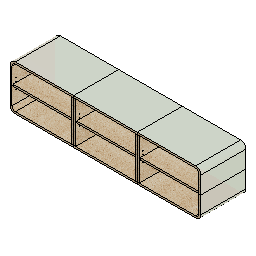
model (Autodesk Fusion 360 design; units mm, degrees)
Autodesk Fusion 360 part; units mm, degrees
note: some values were not read from the file. Chosen so that the rebuilt part matches the saved one: which bodies a step acts on; a side.
sketch "front" plane through (0, 0, 0) normal (0, 1, 0) x (1, 0, 0)
  line L0 (0, 0) -> (1800, 0) construction
  line L1 (1800, 0) -> (1800, -425) construction
  line L2 (1800, -425) -> (0, -425) construction
  line L3 (0, -425) -> (0, 0) construction
  arc A0 (0, -375) -> (50, -425) centre (50, -375) ccw
  arc A1 (50, 0) -> (0, -50) centre (50, -50) ccw
  arc A2 (1800, -50) -> (1750, 0) centre (1750, -50) ccw
  arc A3 (1750, -425) -> (1800, -375) centre (1750, -375) ccw
  line L4 (600, -425) -> (600, 0)
  line L5 (1200, -425) -> (1200, 0)
  line L6 (0, -212.5) -> (600, -212.5) construction
  line L7 (600, -212.5) -> (1200, -212.5) construction
  line L8 (1800, -212.5) -> (1200, -212.5) construction
  line L9 (50, -425) -> (1750, -425)
  line L10 (1800, -375) -> (1800, -50)
  line L11 (1750, 0) -> (50, 0)
  line L12 (0, -50) -> (0, -375)
  arc A4 (1750, -407) -> (1782, -375) centre (1750, -375) ccw
  line L13 (1782, -375) -> (1782, -50)
  arc A5 (1782, -50) -> (1750, -18) centre (1750, -50) ccw
  line L14 (1750, -18) -> (50, -18)
  arc A6 (50, -18) -> (18, -50) centre (50, -50) ccw
  line L15 (18, -50) -> (18, -375)
  arc A7 (18, -375) -> (50, -407) centre (50, -375) ccw
  line L16 (50, -407) -> (1750, -407)
  line L17 (600, -407) -> (600, -425)
  line L18 (1200, -407) -> (1200, -425)
  line L19 (1200, -18) -> (1200, 0)
  line L20 (600, 0) -> (600, -18)
  line L21 (0, -212.5) -> (18, -212.5)
  line L22 (1782, -212.5) -> (1800, -212.5)
  line L23 (582, -407) -> (582, -18)
  line L24 (618, -407) -> (618, -18)
  line L25 (582, -407) -> (600, -212.5) construction
  line L26 (618, -407) -> (600, -212.5) construction
  line L27 (1182, -407) -> (1182, -18)
  line L28 (1218, -407) -> (1218, -18)
  line L29 (18, -221.5) -> (582, -221.5)
  line L30 (18, -203.5) -> (582, -203.5)
  line L31 (18, -221.5) -> (300, -212.5) construction
  line L32 (18, -203.5) -> (300, -212.5) construction
  line L33 (618, -221.5) -> (1182, -221.5)
  line L34 (618, -203.5) -> (1182, -203.5)
  line L35 (1218, -221.5) -> (1782, -221.5)
  line L36 (1218, -203.5) -> (1782, -203.5)
  line L37 (50, 0) -> (50, 18)
  line L38 (50, 18) -> (1750, 18)
  line L39 (1750, 18) -> (1750, 0)
  line L40 (900, 18) -> (900, 0) construction
  dimension "d4" = 425
  dimension "d5" = 1800
  dimension "d6" = 50
  dimension "d9" = 36
  dimension "d12" = 600
  dimension "d13" = 0
  dimension "d14" = 18
  dimension "d23" = 50
  dimension "d24" = 18
  constraint horizontal L0
  constraint vertical L1
  constraint horizontal L2
  constraint vertical L3
  constraint coincident L0.start L3.end
  constraint tangent L2 A0
  constraint coincident L2 A0.end
  constraint coincident L3 A0.start
  constraint tangent L0 A1
  constraint coincident L0 A1.start
  constraint coincident L3 A1.end
  constraint tangent L0 A2
  constraint coincident L1 A2.start
  constraint coincident L0 A2.end
  constraint tangent L2 A3
  constraint coincident L2 A3.start
  constraint coincident L1 A3.end
  constraint tangent L3 A0
  constraint tangent L3 A1
  constraint tangent L1 A2
  constraint tangent L1 A3
  constraint equal A0 A1
  constraint equal A1 A2
  constraint equal A2 A3
  constraint coincident L2 L4.start
  constraint coincident L0 L4.end
  constraint coincident L2 L5.start
  constraint coincident L0 L5.end
  constraint midpoint L3 L6.start
  constraint midpoint L4 L6.end
  constraint midpoint L5 L7.end
  constraint midpoint L1 L8.start
  constraint vertical L4
  constraint vertical L5
  constraint equal L6 L7
  constraint equal L7 L8
  constraint coincident L4 L17.start
  constraint coincident L16 L17.start
  constraint coincident L16 L18.start
  constraint coincident L5 L18.start
  constraint coincident L14 L19.start
  constraint coincident L5 L19.start
  constraint coincident L14 L20.end
  constraint coincident L4 L20.end
  constraint midpoint L15 L21.end
  constraint midpoint L13 L22.start
  constraint coincident L16 L23.start
  constraint coincident L14 L23.end
  constraint coincident L16 L24.start
  constraint coincident L14 L24.end
  constraint vertical L23
  constraint vertical L24
  constraint equal L25 L26
  constraint coincident L15 L29.start
  constraint coincident L23 L29.end
  constraint coincident L15 L30.start
  constraint coincident L23 L30.end
  constraint horizontal L29
  constraint horizontal L30
  constraint midpoint L6 L31.end
  constraint equal L31 L32
  constraint coincident L24 L33.start
  constraint coincident L27 L33.end
  constraint coincident L24 L34.start
  constraint coincident L27 L34.end
  constraint coincident L28 L35.start
  constraint coincident L13 L35.end
  constraint coincident L28 L36.start
  constraint coincident L13 L36.end
  constraint collinear L29 L33
  constraint collinear L33 L35
  constraint collinear L30 L34
  constraint collinear L34 L36
  constraint coincident L11 A2.end
  constraint vertical L37
  constraint horizontal L38
  constraint vertical L39
  constraint midpoint L38 L40.start
  constraint midpoint L0 L40.end
  constraint vertical L40
  measures "d4" distance of L0.start L2.end
  measures "d5" distance of L0.start L0.end
  measures "d6" radius of A0
  measures "d9" distance of L23 L24
  measures "d14" distance of L29.start L30.start
  measures "d23" horizontal distance of L0.start L37.end
  measures "d24" distance of A1.start L37.end
extrude "Extrude1" add sketch "front" along normal blind 425 contours A0 L4 L9 L12 L15 A7 L16 L17 L21 | A3 L5 L9 L10 A4 L13 L16 L18 L22 | L4 L5 L11 L14 L19 L20 | L24 L27 L33 L34 makes body 1 at (1000, 141.6667, 0) makes body 2 at (1383.3333, 141.6667, 407) makes body 3 at (233.3333, 141.6667, 407) makes body 4 at (806, 283.3333, 203.5)
extrude "Extrude2" add sketch "front" along normal blind 425 separate body contours A1 L4 L11 L12 L14 A6 L15 L20 L21 | L4 L5 L9 L16 L17 L18 | A2 L5 L10 L11 L13 A5 L14 L19 L22 makes body 5 at (416.6667, 141.6667, 0) makes body 6 at (800, 141.6667, 407) makes body 7 at (1566.6667, 141.6667, 0)
extrude "Extrude3" add sketch "front" along normal blind 425 separate body contours L15 L23 L29 L30 | L4 L14 L16 L24 | L5 L14 L16 L27 | L13 L28 L35 L36 makes body 8 at (206, 283.3333, 203.5) makes body 9 at (1406, 141.6667, 203.5) makes body 10 at (600, 141.6667, 277.3333) makes body 11 at (1182, 283.3333, 277.3333)
extrude "Extrude4" add sketch "front" along normal blind 425 separate body contours L4 L14 L16 L23 | L5 L14 L16 L28 makes body 12 at (1200, 283.3333, 277.3333) makes body 13 at (582, 283.3333, 277.3333)
extrude "Extrude5" add sketch "front" along normal up to surface (405 mm away) from surface at 20 separate body contours L11 L37 L38 L39 makes body 14
fillet "Fillet1" radius 50 4 edges at (50, 20, -9) (50, 425, -9) (1750, 20, -9) (1750, 425, -9) on bodies 14
sketch "base" plane through (0, 0, -18) normal (0, 0, -1) x (1, 0, 0)
  line L0 (100, -425) -> (1700, -425)
  line L1 (1750, -375) -> (1750, -70)
  line L2 (1700, -20) -> (100, -20)
  line L3 (50, -70) -> (50, -375)
  arc A0 (1700, -425) -> (1750, -375) centre (1700, -375) ccw
  arc A1 (1750, -70) -> (1700, -20) centre (1700, -70) ccw
  arc A2 (100, -20) -> (50, -70) centre (100, -70) ccw
  arc A3 (50, -375) -> (100, -425) centre (100, -375) ccw
  line L4 (100, -393) -> (1700, -393)
  arc A4 (1700, -393) -> (1718, -375) centre (1700, -375) ccw
  line L5 (1718, -375) -> (1718, -70)
  arc A5 (1718, -70) -> (1700, -52) centre (1700, -70) ccw
  line L6 (1700, -52) -> (100, -52)
  arc A6 (100, -52) -> (82, -70) centre (100, -70) ccw
  line L7 (82, -70) -> (82, -375)
  arc A7 (82, -375) -> (100, -393) centre (100, -375) ccw
  line L8 (568, -52) -> (568, -393)
  line L9 (632, -52) -> (632, -393)
  line L10 (1168, -52) -> (1168, -393)
  line L11 (1232, -52) -> (1232, -393)
  line L12 (568, -52) -> (600, 0) construction
  line L13 (600, 0) -> (632, -52) construction
  line L14 (1168, -52) -> (1200, 0) construction
  line L15 (1200, 0) -> (1232, -52) construction
  line L16 (114, -20) -> (114, -425)
  line L17 (1686, -20) -> (1686, -425)
  line L18 (600, 0) -> (600, -425)
  line L19 (1200, 0) -> (1200, -425)
  point P0 (600, 0)
  point P1 (1200, 0)
  dimension "d33" = -32
  dimension "d38" = 64
  dimension "d39" = 64
  dimension "d108" = 64
  dimension "d109" = 64
  constraint coincident L6 L8.start
  constraint coincident L4 L8.end
  constraint coincident L6 L9.start
  constraint coincident L4 L9.end
  constraint coincident L6 L10.start
  constraint coincident L4 L10.end
  constraint coincident L6 L11.start
  constraint coincident L4 L11.end
  constraint vertical L8
  constraint vertical L9
  constraint vertical L10
  constraint vertical L11
  constraint coincident P0 L12.end
  constraint coincident P1 L14.end
  constraint equal L12 L13
  constraint equal L14 L15
  constraint coincident L2 L16.start
  constraint coincident L0 L16.end
  constraint vertical L16
  constraint coincident L2 L17.start
  constraint coincident L0 L17.end
  constraint vertical L17
  constraint coincident L0 L18.end
  constraint coincident L0 L19.end
  constraint vertical L18
  constraint vertical L19
  measures "d38" distance of L8.start L9.start
  measures "d39" distance of L10.start L11.start
  measures "d108" horizontal distance of L3.start L16.start
  measures "d109" horizontal distance of L1.end L17.start
extrude "Extrude6" add sketch "base" against normal up to surface (18 mm away) separate body contours L0 L2 L3 A2 A3 L4 L6 A6 L7 A7 L16 | L4 L6 A6 L7 A7 L16 | L4 L6 L9 L18 | L4 L6 L8 L18 | L0 L1 L2 A0 A1 L4 A4 L5 A5 L6 L17 | L4 L6 L11 L19 | L4 L6 L10 L19 | L4 A4 L5 A5 L6 L17 makes body 15 at (1707.3333, 171.6667, -18) makes body 16 at (1189.3333, 165.6667, -18) makes body 17 at (92.6667, 273.3333, -18) makes body 18 at (589.3333, 279.3333, -18)
extrude "Extrude8" add sketch "base" against normal up to surface (18 mm away) separate body contours L0 L4 L16 L18 | L0 L4 L17 L19 | L2 L6 L16 L18 | L2 L6 L17 L19 makes body 19 at (438, 41.3333, -18) makes body 20 at (1362, 403.6667, -18) makes body 21 at (276, 403.6667, -18) makes body 22 at (1524, 41.3333, -18)
extrude "Extrude14" add sketch "base" against normal up to surface (18 mm away) separate body contours L0 L4 L18 L19 | L2 L6 L18 L19 makes body 23 at (1000, 30.6667, -18) makes body 24 at (800, 414.3333, -18)
move_face "OffsetFaces1" offset -18 3 faces at (806, 425, 209.5) (1406, 425, 209.5) (206, 425, 209.5) on bodies 4 8 9
sketch "back rabbet" plane through (0, 0, 0) normal (0, 1, 0) x (1, 0, 0)
  line L0 (18, -50) -> (18, -375)
  arc A0 (18, -375) -> (50, -407) centre (50, -375) ccw
  line L1 (50, -407) -> (1750, -407)
  line L2 (582, -407) -> (582, -18)
  line L3 (1750, -18) -> (50, -18)
  arc A1 (50, -18) -> (18, -50) centre (50, -50) ccw
  line L4 (618, -407) -> (618, -18)
  line L5 (1182, -407) -> (1182, -18)
  line L6 (1218, -407) -> (1218, -18)
  arc A2 (1750, -407) -> (1782, -375) centre (1750, -375) ccw
  line L7 (1782, -375) -> (1782, -50)
  arc A3 (1782, -50) -> (1750, -18) centre (1750, -50) ccw
  line L8 (1788.35, -375) -> (1788.35, -50)
  arc A4 (1788.35, -50) -> (1750, -11.65) centre (1750, -50) ccw
  line L9 (1750, -11.65) -> (50, -11.65)
  arc A5 (50, -11.65) -> (11.65, -50) centre (50, -50) ccw
  line L10 (11.65, -50) -> (11.65, -375)
  arc A6 (11.65, -375) -> (50, -413.35) centre (50, -375) ccw
  line L11 (50, -413.35) -> (1750, -413.35)
  arc A7 (1750, -413.35) -> (1788.35, -375) centre (1750, -375) ccw
  line L12 (588.35, -413.35) -> (588.35, -11.65)
  line L13 (611.65, -11.65) -> (611.65, -413.35)
  line L14 (900, -413.35) -> (900, -11.65) construction
  line L15 (1211.65, -413.35) -> (1211.65, -11.65)
  line L16 (1188.35, -11.65) -> (1188.35, -413.35)
  dimension "d73" = 6.35
  dimension "d74" = 6.35
  dimension "d75" = 6.35
  constraint coincident L11 L12.start
  constraint coincident L9 L12.end
  constraint coincident L9 L13.start
  constraint coincident L11 L13.end
  constraint vertical L12
  constraint vertical L13
  constraint midpoint L11 L14.start
  constraint midpoint L9 L14.end
  constraint symmetric L12.start L14 L15.start
  constraint symmetric L12.end L14 L15.end
  constraint symmetric L13.start L14 L16.start
  constraint symmetric L13.end L14 L16.end
  measures "d74" horizontal distance of L2.start L12.start
  measures "d75" horizontal distance of L4.start L13.end
extrude "Extrude12" cut sketch "back rabbet" against normal blind 18 from surface at 425 contours L0 A0 L1 L3 A1 L9 A5 L10 A6 L11 L12 | L1 L2 L3 L12 | L3 L9 L13 L16 | L1 L3 L4 L13 | L1 L11 L13 L16 | L1 L3 L5 L16 | L1 L3 A2 L7 A3 L8 A4 L9 L11 A7 L15 | L1 L3 L6 L15 bodies 1 2 3 5 6 7 10 11 13 12
sketch "shelf pins" plane through (1218, 0, 0) normal (1, 0, 0) x (0, 1, 0)
  line L0 (407, 18) -> (407, 407)
  line L1 (407, 407) -> (0, 407)
  line L2 (0, 407) -> (0, 18)
  line L3 (0, 18) -> (407, 18)
  line L4 (37, 407) -> (37, 18) construction
  line L5 (370, 407) -> (370, 18) construction
  line L6 (0, 375) -> (407, 375)
  line L7 (0, 50) -> (407, 50)
  line L8 (0, 310) -> (407, 310) construction
  line L9 (0, 115) -> (407, 115) construction
  circle A0 centre (37, 199.5312) radius 3.9688
  circle A1 centre (37, 135.5312) radius 3.9688 construction
  circle A2 centre (37, 167.5312) radius 3.9688
  circle A3 centre (37, 231.5312) radius 3.9688
  circle A4 centre (37, 263.5312) radius 3.9688
  circle A5 centre (370, 135.5312) radius 3.9688 construction
  circle A6 centre (370, 167.5312) radius 3.9688
  circle A7 centre (370, 199.5312) radius 3.9688
  circle A8 centre (370, 231.5312) radius 3.9688
  circle A9 centre (370, 263.5312) radius 3.9688
  point P0 (37, 212.5)
  dimension "d110" = 37
  dimension "d111" = 37
  dimension "d112" = 65
  dimension "d113" = 65
  dimension "d114" = 7.9375
  dimension "d117" = 333
  dimension "d118" = 32
  dimension "d119" = 407
  dimension "d120" = 12.9688
  dimension "d124" = 52.5313
  dimension "d125" = 149.5312
  dimension "d126" = 46.4688
  dimension "d127" = 143.4688
  constraint coincident L1 L4.start
  constraint coincident L3 L4.end
  constraint vertical L4
  constraint coincident L1 L5.start
  constraint coincident L3 L5.end
  constraint vertical L5
  constraint coincident L2 L8.start
  constraint coincident L0 L8.end
  constraint coincident L2 L9.start
  constraint coincident L0 L9.end
  constraint horizontal L9
  constraint horizontal L8
  constraint coincident L4 A2.centre
  constraint midpoint L4 P0
  measures "d110" distance of L2 L4
  measures "d111" distance of L0.end L5.start
  measures "d112" distance of L6.start L8.start
  measures "d113" distance of L7.start L9.start
  measures "d114" diameter of A0
  measures "d119" distance of L6.start L6.end
  measures "d120" distance of A0.centre P0
  measures "d124" vertical distance of L9.end A6.centre
  measures "d125" distance of L3 A6.centre
  measures "d126" vertical distance of L8.end A9.centre
  measures "d127" vertical distance of L0.end A9.centre
extrude "Extrude16" cut sketch "shelf pins" along normal up to surface (573 mm away) and the other way up to surface (1209 mm away) contours A0 | A2 | A3 | A4 | A6 | A7 | A8 | A9 bodies 2 3 5 7 10 11 13 12
extrude "Extrude13" add sketch "back rabbet" along normal up to surface (18 mm away) from surface at 407 separate body contours L0 A0 L1 L2 L3 A1 | L0 A0 L1 L3 A1 L9 A5 L10 A6 L11 L12 | L1 L2 L3 L12 | L3 L9 L13 L16 | L1 L3 L4 L13 | L1 L11 L13 L16 | L1 L3 L4 L5 | L1 L3 L5 L16 | L1 L3 A2 L7 A3 L8 A4 L9 L11 A7 L15 | L1 L3 L6 L15 | L1 L3 L6 A2 L7 A3 makes body 25 at (229.45, 407, 145.55) makes body 26 at (1391.1, 407, 145.55) makes body 27 at (803.8833, 407, 279.45)
move_face "OffsetFaces8" offset -10 3 faces at (1406, 0, 209.5) (206, 0, 209.5) (806, 0, 209.5) on bodies 4 8 9
sketch "cable holes" plane through (0, 425, 0) normal (0, 1, 0) x (-1, 0, 0)
  line L0 (-1188.35, 413.35) -> (-1188.35, 11.65)
  line L1 (-1188.35, 11.65) -> (-611.65, 11.65)
  line L2 (-611.65, 11.65) -> (-611.65, 413.35)
  line L3 (-611.65, 413.35) -> (-1188.35, 413.35)
  line L4 (-1182, 407) -> (-618, 407) construction
  line L5 (-618, 407) -> (-618, 18) construction
  line L6 (-618, 18) -> (-1182, 18) construction
  line L7 (-1182, 18) -> (-1182, 407) construction
  line L8 (-1057.48, 183.14) -> (-742.52, 183.14) construction
  line L9 (-742.52, 183.14) -> (-742.52, 38.36) construction
  line L10 (-742.52, 38.36) -> (-1057.48, 38.36) construction
  line L11 (-1057.48, 38.36) -> (-1057.48, 183.14) construction
  line L12 (-1182, 203.5) -> (-1057.48, 183.14) construction
  line L13 (-1057.48, 38.36) -> (-1182, 18) construction
  line L14 (-742.52, 38.36) -> (-618, 18) construction
  line L15 (-900, 183.14) -> (-900, 38.36) construction
  line L16 (-1135.74, 167.14) -> (-1135.74, 54.36)
  arc A0 (-1135.74, 54.36) -> (-1103.74, 54.36) centre (-1119.74, 54.36) ccw
  line L17 (-1103.74, 54.36) -> (-1103.74, 167.14)
  arc A1 (-1103.74, 167.14) -> (-1135.74, 167.14) centre (-1119.74, 167.14) ccw
  line L18 (-1119.74, 183.14) -> (-1119.74, 38.36) construction
  line L19 (-1057.48, 58.36) -> (-1057.48, 163.14)
  arc A2 (-1037.48, 183.14) -> (-1057.48, 163.14) centre (-1037.48, 163.14) ccw
  line L20 (-1037.48, 183.14) -> (-762.52, 183.14)
  arc A3 (-742.52, 163.14) -> (-762.52, 183.14) centre (-762.52, 163.14) ccw
  line L21 (-742.52, 163.14) -> (-742.52, 58.36)
  arc A4 (-762.52, 38.36) -> (-742.52, 58.36) centre (-762.52, 58.36) ccw
  line L22 (-762.52, 38.36) -> (-1037.48, 38.36)
  arc A5 (-1057.48, 58.36) -> (-1037.48, 38.36) centre (-1037.48, 58.36) ccw
  line L23 (-1119.74, 110.75) -> (-1057.48, 110.75) construction
  line L24 (-1119.74, 110.75) -> (-1182, 110.75) construction
  line L25 (-618, 203.5) -> (-1182, 203.5) construction
  line L26 (-1119.74, 183.14) -> (-1057.48, 183.14) construction
  line L27 (-664.26, 167.14) -> (-664.26, 54.36)
  arc A6 (-696.26, 54.36) -> (-664.26, 54.36) centre (-680.26, 54.36) ccw
  arc A7 (-664.26, 167.14) -> (-696.26, 167.14) centre (-680.26, 167.14) ccw
  line L28 (-696.26, 54.36) -> (-696.26, 167.14)
  point P0 (-618, 18)
  point P1 (-1182, 18)
  point P2 (-1182, 407)
  point P3 (-618, 407)
  point P4 (-618, 203.5)
  point P5 (-1182, 203.5)
  dimension "d134" = 314.96
  dimension "d135" = 144.78
  dimension "d136" = 32
  dimension "d137" = 20
  constraint horizontal L4
  constraint vertical L5
  constraint horizontal L6
  constraint vertical L7
  constraint coincident P0 L5.end
  constraint coincident P2 L4.start
  constraint horizontal L8
  constraint vertical L9
  constraint horizontal L10
  constraint vertical L11
  constraint coincident P5 L12.start
  constraint coincident P1 L6.end
  constraint equal L13 L14
  constraint equal L12 L13
  constraint midpoint L8 L15.start
  constraint midpoint L10 L15.end
  constraint tangent L16 A0
  constraint tangent A0 L17
  constraint parallel L16 L17
  constraint tangent L17 A1
  constraint tangent L16 A1
  constraint midpoint A1 L18.start
  constraint midpoint A0 L18.end
  constraint vertical L18
  constraint coincident L11 L19.start
  constraint coincident L11 L19.end
  constraint coincident L8 A2.start
  constraint tangent L19 A2
  constraint coincident L8 L20.end
  constraint coincident L9 A3.start
  constraint tangent L20 A3
  constraint coincident L9 L21.end
  constraint coincident L10 A4.start
  constraint tangent L21 A4
  constraint coincident L10 L22.end
  constraint parallel L10 L22
  constraint tangent L22 A5
  constraint tangent A2 L20
  constraint tangent A3 L21
  constraint tangent A4 L22
  constraint tangent L19 A5
  constraint equal A2 A5
  constraint equal A2 A3
  constraint equal A4 A5
  constraint midpoint L18 L23.start
  constraint midpoint L11 L23.end
  constraint coincident L7 L24.end
  constraint equal L23 L24
  constraint horizontal L24
  constraint horizontal L23
  constraint coincident P4 L25.start
  constraint horizontal L26
  constraint symmetric L15 L16.start L27.start
  constraint symmetric L15 L16.end L27.end
  constraint symmetric L15 A0.end A6.start
  constraint symmetric L15 L17.end A7.end
  constraint symmetric L15 A0 A6
  constraint symmetric L15 A1 A7
  measures "d134" distance of L9.end L10.end
  measures "d135" distance of L8 L10
  measures "d136" distance of L16.end A0.end
  measures "d137" radius of A5
extrude "Extrude17" add sketch "cable holes" against normal blind 24.4 from surface at -18 separate body contours L19 A2 L20 A3 L21 A4 L22 A5 makes body 28
extrude "Extrude18" cut sketch "cable holes" against normal up to surface (18 mm away) contours L16 A0 L17 A1 | L27 A6 A7 L28 bodies 27
sketch "door grid" plane through (0, 0, 0) normal (0, 1, 0) x (1, 0, 0)
  arc A0 (0, -375) -> (50, -425) centre (50, -375) ccw
  line L0 (50, -425) -> (600, -425)
  line L1 (600, -425) -> (1200, -425)
  line L2 (1200, -425) -> (1750, -425)
  arc A1 (1750, -425) -> (1800, -375) centre (1750, -375) ccw
  line L3 (1800, -375) -> (1800, -212.5)
  line L4 (1800, -212.5) -> (1800, -50)
  arc A2 (1800, -50) -> (1750, 0) centre (1750, -50) ccw
  line L5 (1750, 0) -> (1200, 0)
  line L6 (1200, 0) -> (600, 0)
  line L7 (600, 0) -> (50, 0)
  arc A3 (50, 0) -> (0, -50) centre (50, -50) ccw
  line L8 (0, -50) -> (0, -212.5)
  line L9 (0, -212.5) -> (0, -375)
  line L10 (40.625, -212.5) -> (40.625, -375)
  arc A4 (40.625, -375) -> (50, -384.375) centre (50, -375) ccw
  line L11 (50, -384.375) -> (600, -384.375)
  line L12 (600, -384.375) -> (1200, -384.375)
  line L13 (1200, -384.375) -> (1750, -384.375)
  arc A5 (1750, -384.375) -> (1759.375, -375) centre (1750, -375) ccw
  line L14 (1759.375, -375) -> (1759.375, -212.5)
  line L15 (1759.375, -212.5) -> (1759.375, -50)
  arc A6 (1759.375, -50) -> (1750, -40.625) centre (1750, -50) ccw
  line L16 (1750, -40.625) -> (1200, -40.625)
  line L17 (1200, -40.625) -> (600, -40.625)
  line L18 (600, -40.625) -> (50, -40.625)
  arc A7 (50, -40.625) -> (40.625, -50) centre (50, -50) ccw
  line L19 (40.625, -50) -> (40.625, -212.5)
  line L20 (40.625, -212.5) -> (1759.375, -212.5)
  line L21 (212.5, -384.375) -> (212.5, -40.625)
  line L22 (556.25, -384.375) -> (556.25, -40.625)
  line L23 (900, -384.375) -> (900, -40.625)
  line L24 (1243.75, -384.375) -> (1243.75, -40.625)
  line L25 (1415.625, -384.375) -> (1415.625, -40.625)
  line L26 (384.375, -384.375) -> (384.375, -40.625)
  line L27 (1071.875, -384.375) -> (1071.875, -40.625)
  line L28 (1587.5, -384.375) -> (1587.5, -40.625)
  line L29 (40.625, -293.75) -> (212.5, -293.75) construction
  line L30 (384.375, -293.75) -> (212.5, -293.75) construction
  line L31 (384.375, -293.75) -> (556.25, -293.75) construction
  line L32 (556.25, -293.75) -> (728.125, -293.75) construction
  line L33 (728.125, -384.375) -> (728.125, -40.625)
  line L34 (728.125, -293.75) -> (900, -293.75) construction
  line L35 (900, -293.75) -> (1071.875, -293.75) construction
  line L36 (1071.875, -293.75) -> (1243.75, -293.75) construction
  line L37 (1243.75, -293.75) -> (1415.625, -293.75) construction
  line L38 (1415.625, -293.75) -> (1587.5, -293.75) construction
  line L39 (1587.5, -293.75) -> (1759.375, -293.75) construction
  dimension "d42" = -40.625
  dimension "d45" = 343.75
  dimension "d46" = 1718.75
  dimension "d48" = 171.875
  constraint horizontal L20
  constraint coincident L11 L21.start
  constraint coincident L18 L21.end
  constraint coincident L11 L22.start
  constraint coincident L18 L22.end
  constraint coincident L12 L23.start
  constraint coincident L17 L23.end
  constraint coincident L12 L24.start
  constraint coincident L17 L24.end
  constraint coincident L16 L25.end
  constraint coincident L13 L25.start
  constraint coincident L11 L26.start
  constraint coincident L18 L26.end
  constraint coincident L17 L27.end
  constraint coincident L13 L28.start
  constraint coincident L16 L28.end
  constraint coincident L12 L27.start
  constraint vertical L21
  constraint vertical L26
  constraint vertical L22
  constraint vertical L23
  constraint vertical L27
  constraint vertical L24
  constraint vertical L25
  constraint vertical L28
  constraint midpoint L10 L29.start
  constraint coincident L21 L29.end
  constraint perpendicular L21 L29
  constraint coincident L26 L30.start
  constraint coincident L22 L31.end
  constraint coincident L12 L33.start
  constraint coincident L17 L33.end
  constraint vertical L33
  constraint coincident L32.end L33
  constraint coincident L23 L34.end
  constraint coincident L27 L35.end
  constraint coincident L24 L36.end
  constraint coincident L25 L37.end
  constraint coincident L28 L38.end
  constraint midpoint L14 L39.end
  constraint horizontal L30
  constraint horizontal L31
  constraint horizontal L32
  constraint horizontal L34
  constraint horizontal L35
  constraint horizontal L36
  constraint horizontal L37
  constraint horizontal L38
  constraint horizontal L39
  constraint equal L29 L30
  constraint equal L30 L31
  constraint equal L31 L32
  constraint equal L32 L34
  constraint equal L34 L35
  constraint equal L35 L36
  constraint equal L36 L37
  constraint equal L37 L38
  constraint equal L38 L39
  measures "d45" distance of L11 L18
  measures "d46" distance of L10 L14
  measures "d48" distance of L21 L26
extrude "Extrude9" [rolled back] taper angle 0
extrude "Extrude10" [rolled back] taper angle 0
sketch "door pattern" plane through (0, -16, 0) normal (0, -1, 0) x (1, 0, 0)
  line L0 (40.625, 375) -> (40.625, 50)
  arc A0 (40.625, 50) -> (50, 40.625) centre (50, 50) ccw
  line L1 (50, 40.625) -> (1750, 40.625)
  arc A1 (1750, 40.625) -> (1759.375, 50) centre (1750, 50) ccw
  line L2 (1759.375, 50) -> (1759.375, 375)
  arc A2 (1759.375, 375) -> (1750, 384.375) centre (1750, 375) ccw
  line L3 (1750, 384.375) -> (50, 384.375)
  arc A3 (50, 384.375) -> (40.625, 375) centre (50, 375) ccw
  line L4 (40.625, 212.5) -> (212.5, 212.5)
  line L5 (212.5, 212.5) -> (212.5, 384.375)
  line L6 (212.5, 384.375) -> (40.625, 384.375)
  line L7 (40.625, 384.375) -> (40.625, 212.5)
  line L8 (126.5625, 212.5) -> (126.5625, 40.625) construction
  line L9 (40.625, 368.75) -> (56.25, 368.75) construction
  line L10 (56.25, 368.75) -> (56.25, 384.375) construction
  line L11 (56.25, 368.75) -> (71.875, 368.75) construction
  line L12 (71.875, 368.75) -> (71.875, 384.375) construction
  line L13 (71.875, 368.75) -> (87.5, 368.75) construction
  line L14 (87.5, 368.75) -> (87.5, 384.375) construction
  line L15 (87.5, 368.75) -> (103.125, 368.75) construction
  line L16 (103.125, 368.75) -> (103.125, 384.375) construction
  line L17 (103.125, 368.75) -> (118.75, 368.75) construction
  line L18 (118.75, 368.75) -> (118.75, 384.375) construction
  line L19 (118.75, 368.75) -> (134.375, 368.75) construction
  line L20 (134.375, 368.75) -> (134.375, 384.375) construction
  line L21 (134.375, 368.75) -> (150, 368.75) construction
  line L22 (150, 368.75) -> (150, 384.375) construction
  line L23 (150, 368.75) -> (165.625, 368.75) construction
  line L24 (165.625, 368.75) -> (165.625, 384.375) construction
  line L25 (165.625, 368.75) -> (181.25, 368.75) construction
  line L26 (181.25, 368.75) -> (181.25, 384.375) construction
  line L27 (181.25, 368.75) -> (196.875, 368.75) construction
  line L28 (196.875, 368.75) -> (196.875, 384.375) construction
  line L29 (196.875, 368.75) -> (212.5, 368.75) construction
  line L30 (212.5, 368.75) -> (212.5, 384.375) construction
  line L31 (40.625, 353.125) -> (56.25, 353.125) construction
  line L32 (56.25, 353.125) -> (56.25, 368.75) construction
  line L33 (56.25, 353.125) -> (71.875, 353.125) construction
  line L34 (71.875, 353.125) -> (71.875, 368.75) construction
  line L35 (71.875, 353.125) -> (87.5, 353.125) construction
  line L36 (87.5, 353.125) -> (87.5, 368.75) construction
  line L37 (87.5, 353.125) -> (103.125, 353.125) construction
  line L38 (103.125, 353.125) -> (103.125, 368.75) construction
  line L39 (103.125, 353.125) -> (118.75, 353.125) construction
  line L40 (118.75, 353.125) -> (118.75, 368.75) construction
  line L41 (118.75, 353.125) -> (134.375, 353.125) construction
  line L42 (134.375, 353.125) -> (134.375, 368.75) construction
  line L43 (134.375, 353.125) -> (150, 353.125) construction
  line L44 (150, 353.125) -> (150, 368.75) construction
  line L45 (150, 353.125) -> (165.625, 353.125) construction
  line L46 (165.625, 353.125) -> (165.625, 368.75) construction
  line L47 (165.625, 353.125) -> (181.25, 353.125) construction
  line L48 (181.25, 353.125) -> (181.25, 368.75) construction
  line L49 (181.25, 353.125) -> (196.875, 353.125) construction
  line L50 (196.875, 353.125) -> (196.875, 368.75) construction
  line L51 (196.875, 353.125) -> (212.5, 353.125) construction
  line L52 (212.5, 353.125) -> (212.5, 368.75) construction
  line L53 (40.625, 337.5) -> (56.25, 337.5) construction
  line L54 (56.25, 337.5) -> (56.25, 353.125) construction
  line L55 (56.25, 337.5) -> (71.875, 337.5) construction
  line L56 (71.875, 337.5) -> (71.875, 353.125) construction
  line L57 (71.875, 337.5) -> (87.5, 337.5) construction
  line L58 (87.5, 337.5) -> (87.5, 353.125) construction
  line L59 (87.5, 337.5) -> (103.125, 337.5) construction
  line L60 (103.125, 337.5) -> (103.125, 353.125) construction
  line L61 (103.125, 337.5) -> (118.75, 337.5) construction
  line L62 (118.75, 337.5) -> (118.75, 353.125) construction
  line L63 (118.75, 337.5) -> (134.375, 337.5) construction
  line L64 (134.375, 337.5) -> (134.375, 353.125) construction
  line L65 (134.375, 337.5) -> (150, 337.5) construction
  line L66 (150, 337.5) -> (150, 353.125) construction
  line L67 (150, 337.5) -> (165.625, 337.5) construction
  line L68 (165.625, 337.5) -> (165.625, 353.125) construction
  line L69 (165.625, 337.5) -> (181.25, 337.5) construction
  line L70 (181.25, 337.5) -> (181.25, 353.125) construction
  line L71 (181.25, 337.5) -> (196.875, 337.5) construction
  line L72 (196.875, 337.5) -> (196.875, 353.125) construction
  line L73 (196.875, 337.5) -> (212.5, 337.5) construction
  line L74 (212.5, 337.5) -> (212.5, 353.125) construction
  line L75 (40.625, 321.875) -> (56.25, 321.875) construction
  line L76 (56.25, 321.875) -> (56.25, 337.5) construction
  line L77 (56.25, 321.875) -> (71.875, 321.875) construction
  line L78 (71.875, 321.875) -> (71.875, 337.5) construction
  line L79 (71.875, 321.875) -> (87.5, 321.875) construction
  line L80 (87.5, 321.875) -> (87.5, 337.5) construction
  line L81 (87.5, 321.875) -> (103.125, 321.875) construction
  line L82 (103.125, 321.875) -> (103.125, 337.5) construction
  line L83 (103.125, 321.875) -> (118.75, 321.875) construction
  line L84 (118.75, 321.875) -> (118.75, 337.5) construction
  line L85 (118.75, 321.875) -> (134.375, 321.875) construction
  line L86 (134.375, 321.875) -> (134.375, 337.5) construction
  line L87 (134.375, 321.875) -> (150, 321.875) construction
  line L88 (150, 321.875) -> (150, 337.5) construction
  line L89 (150, 321.875) -> (165.625, 321.875) construction
  line L90 (165.625, 321.875) -> (165.625, 337.5) construction
  line L91 (165.625, 321.875) -> (181.25, 321.875) construction
  line L92 (181.25, 321.875) -> (181.25, 337.5) construction
  line L93 (181.25, 321.875) -> (196.875, 321.875) construction
  line L94 (196.875, 321.875) -> (196.875, 337.5) construction
  line L95 (196.875, 321.875) -> (212.5, 321.875) construction
  line L96 (212.5, 321.875) -> (212.5, 337.5) construction
  line L97 (40.625, 306.25) -> (56.25, 306.25) construction
  line L98 (56.25, 306.25) -> (56.25, 321.875) construction
  line L99 (56.25, 306.25) -> (71.875, 306.25) construction
  line L100 (71.875, 306.25) -> (71.875, 321.875) construction
  line L101 (71.875, 306.25) -> (87.5, 306.25) construction
  line L102 (87.5, 306.25) -> (87.5, 321.875) construction
  line L103 (87.5, 306.25) -> (103.125, 306.25) construction
  line L104 (103.125, 306.25) -> (103.125, 321.875) construction
  line L105 (103.125, 306.25) -> (118.75, 306.25) construction
  line L106 (118.75, 306.25) -> (118.75, 321.875) construction
  line L107 (118.75, 306.25) -> (134.375, 306.25) construction
  line L108 (134.375, 306.25) -> (134.375, 321.875) construction
  line L109 (134.375, 306.25) -> (150, 306.25) construction
  line L110 (150, 306.25) -> (150, 321.875) construction
  line L111 (150, 306.25) -> (165.625, 306.25) construction
  line L112 (165.625, 306.25) -> (165.625, 321.875) construction
  line L113 (165.625, 306.25) -> (181.25, 306.25) construction
  line L114 (181.25, 306.25) -> (181.25, 321.875) construction
  line L115 (181.25, 306.25) -> (196.875, 306.25) construction
  line L116 (196.875, 306.25) -> (196.875, 321.875) construction
  line L117 (196.875, 306.25) -> (212.5, 306.25) construction
  line L118 (212.5, 306.25) -> (212.5, 321.875) construction
  line L119 (40.625, 290.625) -> (56.25, 290.625) construction
  line L120 (56.25, 290.625) -> (56.25, 306.25) construction
  line L121 (56.25, 290.625) -> (71.875, 290.625) construction
  line L122 (71.875, 290.625) -> (71.875, 306.25) construction
  line L123 (71.875, 290.625) -> (87.5, 290.625) construction
  line L124 (87.5, 290.625) -> (87.5, 306.25) construction
  line L125 (87.5, 290.625) -> (103.125, 290.625) construction
  line L126 (103.125, 290.625) -> (103.125, 306.25) construction
  line L127 (103.125, 290.625) -> (118.75, 290.625) construction
  line L128 (118.75, 290.625) -> (118.75, 306.25) construction
  line L129 (118.75, 290.625) -> (134.375, 290.625) construction
  line L130 (134.375, 290.625) -> (134.375, 306.25) construction
  line L131 (134.375, 290.625) -> (150, 290.625) construction
  line L132 (150, 290.625) -> (150, 306.25) construction
  line L133 (150, 290.625) -> (165.625, 290.625) construction
  line L134 (165.625, 290.625) -> (165.625, 306.25) construction
  line L135 (165.625, 290.625) -> (181.25, 290.625) construction
  line L136 (181.25, 290.625) -> (181.25, 306.25) construction
  line L137 (181.25, 290.625) -> (196.875, 290.625) construction
  line L138 (196.875, 290.625) -> (196.875, 306.25) construction
  line L139 (196.875, 290.625) -> (212.5, 290.625) construction
  line L140 (212.5, 290.625) -> (212.5, 306.25) construction
  line L141 (40.625, 275) -> (56.25, 275) construction
  line L142 (56.25, 275) -> (56.25, 290.625) construction
  line L143 (56.25, 275) -> (71.875, 275) construction
  line L144 (71.875, 275) -> (71.875, 290.625) construction
  line L145 (71.875, 275) -> (87.5, 275) construction
  line L146 (87.5, 275) -> (87.5, 290.625) construction
  line L147 (87.5, 275) -> (103.125, 275) construction
  line L148 (103.125, 275) -> (103.125, 290.625) construction
  line L149 (103.125, 275) -> (118.75, 275) construction
  line L150 (118.75, 275) -> (118.75, 290.625) construction
  line L151 (118.75, 275) -> (134.375, 275) construction
  line L152 (134.375, 275) -> (134.375, 290.625) construction
  line L153 (134.375, 275) -> (150, 275) construction
  line L154 (150, 275) -> (150, 290.625) construction
  line L155 (150, 275) -> (165.625, 275) construction
  line L156 (165.625, 275) -> (165.625, 290.625) construction
  line L157 (165.625, 275) -> (181.25, 275) construction
  line L158 (181.25, 275) -> (181.25, 290.625) construction
  line L159 (181.25, 275) -> (196.875, 275) construction
  line L160 (196.875, 275) -> (196.875, 290.625) construction
  line L161 (196.875, 275) -> (212.5, 275) construction
  line L162 (212.5, 275) -> (212.5, 290.625) construction
  line L163 (40.625, 259.375) -> (56.25, 259.375) construction
  line L164 (56.25, 259.375) -> (56.25, 275) construction
  line L165 (56.25, 259.375) -> (71.875, 259.375) construction
  line L166 (71.875, 259.375) -> (71.875, 275) construction
  line L167 (71.875, 259.375) -> (87.5, 259.375) construction
  line L168 (87.5, 259.375) -> (87.5, 275) construction
  line L169 (87.5, 259.375) -> (103.125, 259.375) construction
  line L170 (103.125, 259.375) -> (103.125, 275) construction
  line L171 (103.125, 259.375) -> (118.75, 259.375) construction
  line L172 (118.75, 259.375) -> (118.75, 275) construction
  line L173 (118.75, 259.375) -> (134.375, 259.375) construction
  line L174 (134.375, 259.375) -> (134.375, 275) construction
  line L175 (134.375, 259.375) -> (150, 259.375) construction
  line L176 (150, 259.375) -> (150, 275) construction
  line L177 (150, 259.375) -> (165.625, 259.375) construction
  line L178 (165.625, 259.375) -> (165.625, 275) construction
  line L179 (165.625, 259.375) -> (181.25, 259.375) construction
  line L180 (181.25, 259.375) -> (181.25, 275) construction
  line L181 (181.25, 259.375) -> (196.875, 259.375) construction
  line L182 (196.875, 259.375) -> (196.875, 275) construction
  line L183 (196.875, 259.375) -> (212.5, 259.375) construction
  line L184 (212.5, 259.375) -> (212.5, 275) construction
  line L185 (40.625, 243.75) -> (56.25, 243.75) construction
  line L186 (56.25, 243.75) -> (56.25, 259.375) construction
  line L187 (56.25, 243.75) -> (71.875, 243.75) construction
  line L188 (71.875, 243.75) -> (71.875, 259.375) construction
  line L189 (71.875, 243.75) -> (87.5, 243.75) construction
  line L190 (87.5, 243.75) -> (87.5, 259.375) construction
  line L191 (87.5, 243.75) -> (103.125, 243.75) construction
  line L192 (103.125, 243.75) -> (103.125, 259.375) construction
  line L193 (103.125, 243.75) -> (118.75, 243.75) construction
  line L194 (118.75, 243.75) -> (118.75, 259.375) construction
  line L195 (118.75, 243.75) -> (134.375, 243.75) construction
  line L196 (134.375, 243.75) -> (134.375, 259.375) construction
  line L197 (134.375, 243.75) -> (150, 243.75) construction
  line L198 (150, 243.75) -> (150, 259.375) construction
  line L199 (150, 243.75) -> (165.625, 243.75) construction
  line L200 (165.625, 243.75) -> (165.625, 259.375) construction
  line L201 (165.625, 243.75) -> (181.25, 243.75) construction
  line L202 (181.25, 243.75) -> (181.25, 259.375) construction
  line L203 (181.25, 243.75) -> (196.875, 243.75) construction
  line L204 (196.875, 243.75) -> (196.875, 259.375) construction
  line L205 (196.875, 243.75) -> (212.5, 243.75) construction
  line L206 (212.5, 243.75) -> (212.5, 259.375) construction
  line L207 (40.625, 228.125) -> (56.25, 228.125) construction
  line L208 (56.25, 228.125) -> (56.25, 243.75) construction
  line L209 (56.25, 228.125) -> (71.875, 228.125) construction
  line L210 (71.875, 228.125) -> (71.875, 243.75) construction
  line L211 (71.875, 228.125) -> (87.5, 228.125) construction
  line L212 (87.5, 228.125) -> (87.5, 243.75) construction
  line L213 (87.5, 228.125) -> (103.125, 228.125) construction
  line L214 (103.125, 228.125) -> (103.125, 243.75) construction
  line L215 (103.125, 228.125) -> (118.75, 228.125) construction
  line L216 (118.75, 228.125) -> (118.75, 243.75) construction
  line L217 (118.75, 228.125) -> (134.375, 228.125) construction
  line L218 (134.375, 228.125) -> (134.375, 243.75) construction
  line L219 (134.375, 228.125) -> (150, 228.125) construction
  line L220 (150, 228.125) -> (150, 243.75) construction
  line L221 (150, 228.125) -> (165.625, 228.125) construction
  line L222 (165.625, 228.125) -> (165.625, 243.75) construction
  line L223 (165.625, 228.125) -> (181.25, 228.125) construction
  line L224 (181.25, 228.125) -> (181.25, 243.75) construction
  line L225 (181.25, 228.125) -> (196.875, 228.125) construction
  line L226 (196.875, 228.125) -> (196.875, 243.75) construction
  line L227 (196.875, 228.125) -> (212.5, 228.125) construction
  line L228 (212.5, 228.125) -> (212.5, 243.75) construction
  line L229 (40.625, 212.5) -> (56.25, 212.5) construction
  line L230 (56.25, 212.5) -> (56.25, 228.125) construction
  line L231 (56.25, 212.5) -> (71.875, 212.5) construction
  line L232 (71.875, 212.5) -> (71.875, 228.125) construction
  line L233 (71.875, 212.5) -> (87.5, 212.5) construction
  line L234 (87.5, 212.5) -> (87.5, 228.125) construction
  line L235 (87.5, 212.5) -> (103.125, 212.5) construction
  line L236 (103.125, 212.5) -> (103.125, 228.125) construction
  line L237 (103.125, 212.5) -> (118.75, 212.5) construction
  line L238 (118.75, 212.5) -> (118.75, 228.125) construction
  line L239 (118.75, 212.5) -> (134.375, 212.5) construction
  line L240 (134.375, 212.5) -> (134.375, 228.125) construction
  line L241 (134.375, 212.5) -> (150, 212.5) construction
  line L242 (150, 212.5) -> (150, 228.125) construction
  line L243 (150, 212.5) -> (165.625, 212.5) construction
  line L244 (165.625, 212.5) -> (165.625, 228.125) construction
  line L245 (165.625, 212.5) -> (181.25, 212.5) construction
  line L246 (181.25, 212.5) -> (181.25, 228.125) construction
  line L247 (181.25, 212.5) -> (196.875, 212.5) construction
  line L248 (196.875, 212.5) -> (196.875, 228.125) construction
  line L249 (196.875, 212.5) -> (212.5, 212.5) construction
  line L250 (212.5, 212.5) -> (212.5, 228.125) construction
  arc A4 (212.5, 368.75) -> (56.25, 212.5) centre (212.5, 212.5) ccw
  arc A5 (212.5, 353.125) -> (71.875, 212.5) centre (212.5, 212.5) ccw
  arc A6 (212.5, 337.5) -> (87.5, 212.5) centre (212.5, 212.5) ccw
  arc A7 (212.5, 321.875) -> (103.125, 212.5) centre (212.5, 212.5) ccw
  arc A8 (212.5, 306.25) -> (118.75, 212.5) centre (212.5, 212.5) ccw
  arc A9 (212.5, 290.625) -> (134.375, 212.5) centre (212.5, 212.5) ccw
  arc A10 (212.5, 275) -> (150, 212.5) centre (212.5, 212.5) ccw
  arc A11 (212.5, 259.375) -> (165.625, 212.5) centre (212.5, 212.5) ccw
  arc A12 (212.5, 243.75) -> (181.25, 212.5) centre (212.5, 212.5) ccw
  arc A13 (212.5, 228.125) -> (196.875, 212.5) centre (212.5, 212.5) ccw
  arc A14 (40.625, 321.875) -> (103.125, 384.375) centre (40.625, 384.375) ccw
  arc A15 (40.625, 337.5) -> (87.5, 384.375) centre (40.625, 384.375) ccw
  arc A16 (40.625, 353.125) -> (71.875, 384.375) centre (40.625, 384.375) ccw
  arc A17 (40.625, 368.75) -> (56.25, 384.375) centre (40.625, 384.375) ccw
  arc A18 (212.5, 384.375) -> (40.625, 212.5) centre (212.5, 212.5) ccw construction
  arc A19 (115.2905, 361.3843) -> (118.75, 384.375) centre (40.625, 384.375) ccw
  arc A20 (130.2236, 356.7861) -> (134.375, 384.375) centre (40.625, 384.375) ccw
  arc A21 (149.6733, 375.9281) -> (150, 384.375) centre (40.625, 384.375) ccw
  arc A22 (165.2517, 374.7214) -> (165.625, 384.375) centre (40.625, 384.375) ccw
  arc A23 (181.2418, 382.8529) -> (181.25, 384.375) centre (40.625, 384.375) ccw
  arc A24 (196.8658, 382.6837) -> (196.875, 384.375) centre (40.625, 384.375) ccw
  line L251 (40.625, 384.375) -> (212.5, 212.5) construction
  arc A25 (115.2905, 361.3843) -> (130.2236, 356.7861) centre (122.7571, 359.0852) ccw
  arc A26 (149.6733, 375.9281) -> (165.2517, 374.7214) centre (157.4625, 375.3247) ccw
  arc A27 (181.2418, 382.8529) -> (196.8658, 382.6837) centre (189.0538, 382.7683) ccw
  arc A28 (40.625, 290.625) -> (68.2139, 294.7764) centre (40.625, 384.375) ccw
  arc A29 (68.2139, 294.7764) -> (63.6157, 309.7095) centre (65.9148, 302.2429) ccw
  arc A30 (40.625, 306.25) -> (63.6157, 309.7095) centre (40.625, 384.375) ccw
  arc A31 (40.625, 275) -> (49.0719, 275.3267) centre (40.625, 384.375) ccw
  arc A32 (40.625, 259.375) -> (50.2786, 259.7483) centre (40.625, 384.375) ccw
  arc A33 (50.2786, 259.7483) -> (49.0719, 275.3267) centre (49.6753, 267.5375) ccw
  arc A34 (40.625, 243.75) -> (42.1471, 243.7582) centre (40.625, 384.375) ccw
  arc A35 (40.625, 228.125) -> (42.3163, 228.1342) centre (40.625, 384.375) ccw
  arc A36 (42.3163, 228.1342) -> (42.1471, 243.7582) centre (42.2317, 235.9462) ccw
  dimension "d54" = 171.875
  dimension "d55" = 15.625
  dimension "d59" = 15.625
  dimension "d60" = -15.625
  constraint horizontal L4
  constraint vertical L5
  constraint horizontal L6
  constraint vertical L7
  constraint coincident L3 L5.end
  constraint coincident L0 L4.start
  constraint equal L4 L5
  constraint midpoint L4 L8.start
  constraint coincident L1 L8.end
  constraint perpendicular L1 L8
  constraint equal L5 L8
  constraint coincident L7 L9.start
  constraint coincident L6 L10.end
  constraint horizontal L9
  constraint vertical L10
  constraint equal L9 L10
  constraint coincident L4.end L5.start
  constraint coincident L6.end L7.start
  constraint tangent A19 A25
  constraint tangent A21 A26
  constraint tangent A23 A27
  constraint tangent A20 A25
  constraint tangent A22 A26
  constraint tangent A24 A27
  constraint coincident A18 A25.centre
  constraint coincident A18 A26.centre
  constraint coincident A18 A27.centre
  constraint symmetric L18.end L251 L97.start
  constraint symmetric L20.end L251 L119.start
  constraint symmetric L22.end L251 L141.start
  constraint symmetric L24.end L251 L163.start
  constraint symmetric L26.end L251 L185.start
  constraint symmetric L28.end L251 L207.start
  constraint symmetric A19.start L251 A29.end
  constraint symmetric A19 L251 A30
  constraint symmetric A20.start L251 A28.end
  constraint symmetric A20 L251 A28
  constraint symmetric A21.start L251 A31.end
  constraint symmetric A21 L251 A31
  constraint symmetric A22.start L251 A32.end
  constraint symmetric A22 L251 A32
  constraint symmetric A23.start L251 A34.end
  constraint symmetric A23 L251 A34
  constraint symmetric A24.start L251 A35.end
  constraint symmetric A24 L251 A35
  constraint symmetric L251 A25 A29
  constraint symmetric L251 A26 A33
  constraint symmetric L251 A27 A36
  measures "d54" distance of L5.end L6.end
  measures "d55" distance of L6.end L10.end
extrude "Extrude11" [rolled back] side1offset 0 taper angle 0
pattern_linear "R-Pattern1" [rolled back] count u 10 u space distance 171.875 v space distance -171.875
combine "Combine1" [rolled back]
move_face "OffsetFaces2" [rolled back] distance 2
move_face "OffsetFaces3" [rolled back]
split "Split1" [rolled back]
split "Split2" [rolled back]
move_face "OffsetFaces4" [rolled back] distance -2
move_face "OffsetFaces5" [rolled back] distance -2
move_face "OffsetFaces6" [rolled back] distance -2
move_face "OffsetFaces7" [rolled back] distance -2
chamfer "Chamfer3" [rolled back] distance 2
hidden bodies 14
equation "depth = 425 mm"
equation "unitWidth = 600 mm"
equation "bendRadius = 50 mm"
equation "d4 = depth"
equation "d5 = unitWidth * 3"
equation "d6 = bendRadius"
equation "d7 = -th"
equation "th = 18 mm"
equation "d9 = 2 * th"
equation "d12 = unitWidth"
equation "d14 = th"
equation "d15 = depth"
equation "d17 = depth"
equation "d19 = depth"
equation "d21 = depth"
equation "d23 = bendRadius"
equation "d34 = -th"
equation "d39 = d38"
equation "d42 = ( -81.25 / 2 ) * 1 mm"
equation "d49 = -th + patternDepth"
equation "d51 = -th"
equation "patternDepth = 2 mm"
equation "d55 = d54 / patternGrid"
equation "patternGrid = 11"
equation "d57 = patternGrid"
equation "d58 = patternGrid"
equation "d59 = d55"
equation "d60 = -d55"
equation "d65 = d54"
equation "d66 = -d54"
equation "d67 = patternDepth"
equation "d72 = -patternDepth"
equation "d73 = 1/4\""
equation "d74 = d73"
equation "d75 = d73"
equation "d77 = -th"
equation "d108 = d38"
equation "d109 = d108"
equation "d111 = d110"
equation "d112 = 45 mm + 20 mm"
equation "d113 = d112"
equation "d114 = 5/16\""
equation "d117 = d119 - 2 * d110"
equation "d120 = th / 2 + d114 / 2"
equation "d128 = -th / 2"
equation "d130 = -th / 2"
equation "d139 = 1 mm - 1\""
named bodies: "door1", "door3", "door2"
